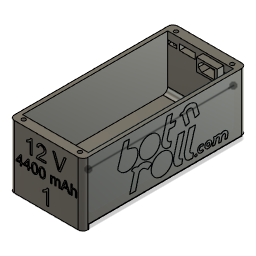
Bateria+Nova (Autodesk Fusion 360 design; units mm, degrees)
Autodesk Fusion 360 part; units mm, degrees
note: some values were not read from the file. Set by a fixed rule: which sketch regions a step uses.
sketch "Esboço1" plane through (0, 0, 0) normal (0, 1, 0) x (1, 0, 0)
  line L0 (0, 0) -> (-76, 0)
  line L1 (-76, 0) -> (-76, 169)
  line L2 (-76, 169) -> (0, 169)
  line L3 (0, 169) -> (0, 0)
  dimension "d1" = 76
  dimension "d2" = 169
  constraint horizontal L0
  constraint vertical L1
  constraint horizontal L2
  constraint vertical L3
  constraint coincident L0.start L3.end
  measures "d1" distance of L0.start L0.end
  measures "d2" distance of L0.start L2.end
extrude "Extrusão1" add sketch "Esboço1" along normal blind 65
sketch "Esboço2" plane through (0, 65, 0) normal (0, 1, 0) x (-1, 0, 0)
  line L0 (0, -169) -> (76, -169)
  line L1 (76, -169) -> (76, 0)
  line L2 (76, 0) -> (0, 0)
  line L3 (0, 0) -> (0, -169)
  line L4 (72, -159.5) -> (4, -159.5)
  line L5 (4, -159.5) -> (4, -9.5)
  line L6 (4, -9.5) -> (72, -9.5)
  line L7 (72, -9.5) -> (72, -159.5)
  dimension "d5" = 4
  dimension "d6" = 4
  dimension "d7" = 150
  dimension "d8" = 9.5
  constraint horizontal L4
  constraint vertical L5
  constraint horizontal L6
  constraint vertical L7
  measures "d5" distance of L1 L7
  measures "d6" distance of L3 L5
  measures "d7" distance of L4.start L6.end
  measures "d8" distance of L2 L6
extrude "Extrusão2" cut sketch "Esboço2" against normal blind 55 contours L4 L5 L6 L7
fillet "Arredondamento1" radius 5 2 edges at (-38, 10, -159.5) (-38, 10, -9.5)
sketch "Esboço3" plane through (-4, 0, 0) normal (-1, 0, 0) x (0, 0, 1)
  arc A0 (-14.5, 10) -> (-9.5, 15) centre (-14.5, 15) ccw
  line L0 (-9.5, 15) -> (-9.5, 65)
  line L1 (-9.5, 65) -> (-159.5, 65)
  line L2 (-159.5, 65) -> (-159.5, 15)
  arc A1 (-159.5, 15) -> (-154.5, 10) centre (-154.5, 15) ccw
  line L3 (-154.5, 10) -> (-14.5, 10)
  line L4 (-159.5, 50) -> (-155, 50)
  line L5 (-155, 50) -> (-9.5, 50)
  dimension "d13" = 40
  constraint coincident L2 L4.start
  constraint perpendicular L2 L4
  constraint coincident L0 L5.end
  constraint perpendicular L0 L5
  measures "d13" distance of L3 L5
sketch "Esboço4" plane through (0, 0, -169) normal (0, 0, -1) x (-1, 0, 0)
  line L0 (0, 0) -> (76, 0)
  line L1 (76, 0) -> (76, 65)
  line L2 (76, 65) -> (0, 65)
  line L3 (0, 65) -> (0, 0)
  line L4 (30.7398, 50) -> (35.5, 54.0801)
  line L5 (35.5, 58.9199) -> (35.5, 54.0801)
  line L6 (30.7398, 63) -> (35.5, 58.9199)
  line L7 (15, 63) -> (30.7398, 63)
  line L8 (15, 63) -> (15, 50)
  line L9 (15, 50) -> (30.7398, 50)
  line L10 (30, 52) -> (33.5, 55)
  line L11 (33.5, 58) -> (33.5, 55)
  line L12 (30, 61) -> (33.5, 58)
  line L13 (17, 61) -> (30, 61)
  line L14 (17, 52) -> (30, 52)
  line L15 (17, 61) -> (17, 52)
  line L16 (43.5, 59.5) -> (59.75, 59.5)
  line L17 (59.75, 59.5) -> (59.75, 53.5)
  line L18 (59.75, 53.5) -> (43.5, 53.5)
  line L19 (43.5, 53.5) -> (43.5, 59.5)
  dimension "d24" = 2
  dimension "d15" = 9
  dimension "d16" = 13
  dimension "d17" = 4.6098
  dimension "d18" = 3
  dimension "d19" = 4.6098
  dimension "d20" = 13
  dimension "d21" = 130.601
  dimension "d22" = 130.601
  dimension "d23" = 139.399
  dimension "d25" = 16.25
  dimension "d26" = 6
  dimension "d27" = 5.5
  dimension "d28" = 15
  dimension "d29" = 10
  dimension "d42" = 2
  constraint horizontal L16
  constraint vertical L17
  constraint horizontal L18
  constraint vertical L19
  measures "d15" distance of L14.start L13.start
  measures "d16" distance of L12.start L13.start
  measures "d17" distance of L11.start L12.start
  measures "d18" distance of L11.start L10.end
  measures "d19" distance of L10.start L10.end
  measures "d20" distance of L10.start L14.start
  measures "d21" angle of L10 L11
  measures "d22" angle of L11 L12
  measures "d23" angle of L12 L13
  measures "d25" distance of L16.start L16.end
  measures "d26" distance of L16.start L18.end
  measures "d27" distance of L2 L16
  measures "d28" distance of L3 L8
  measures "d29" distance of L11 L19
  measures "d42" distance of L2 L7
extrude "Extrusão3" cut sketch "Esboço4" against normal blind 20 contours L10 L11 L12 L13 L14 L15 | L16 L17 L18 L19
sketch "Esboço6" plane through (0, 0, -159.5) normal (0, 0, 1) x (1, 0, 0)
  line L0 (-17, 61) -> (-17, 52)
  line L1 (-17, 52) -> (-30, 52)
  line L2 (-30, 52) -> (-33.5, 55)
  line L3 (-33.5, 55) -> (-33.5, 58)
  line L4 (-33.5, 58) -> (-30, 61)
  line L5 (-30, 61) -> (-17, 61)
  line L6 (-59.75, 53.5) -> (-59.75, 59.5)
  line L7 (-59.75, 59.5) -> (-43.5, 59.5)
  line L8 (-43.5, 59.5) -> (-43.5, 53.5)
  line L9 (-43.5, 53.5) -> (-59.75, 53.5)
  line L10 (-72, 15) -> (-4, 15)
  line L11 (-4, 15) -> (-4, 65)
  line L12 (-4, 65) -> (-72, 65)
  line L13 (-72, 65) -> (-72, 15)
  line L14 (-35.5, 63) -> (-14, 63)
  line L15 (-14, 63) -> (-14, 50)
  line L16 (-14, 50) -> (-35.5, 50)
  line L17 (-35.5, 50) -> (-35.5, 63)
  dimension "d33" = 3
  dimension "d34" = 2
  dimension "d35" = 2
  dimension "d36" = 2
  constraint horizontal L14
  constraint vertical L15
  constraint horizontal L16
  constraint vertical L17
  measures "d33" distance of L0 L15
  measures "d34" distance of L5 L14
  measures "d35" distance of L3 L17
  measures "d36" distance of L1 L16
extrude "Extrusão4" add sketch "Esboço6" along normal blind 6.7 contours L14 L15 L16 L17
sketch "Esboço5" plane through (0, 0, -169) normal (0, 0, -1) x (-1, 0, 0)
  line L0 (15, 63) -> (15, 50.0001)
  line L1 (15, 50.0001) -> (30.7398, 50.0001)
  line L2 (30.7398, 50.0001) -> (35.5, 54.0802)
  line L3 (35.5, 54.0802) -> (35.5, 58.9199)
  line L4 (35.5, 58.9199) -> (30.7398, 63)
  line L5 (30.7398, 63) -> (15, 63)
  line L6 (17, 61) -> (30, 61)
  line L7 (33.5, 58) -> (33.5, 55)
extrude "Extrusão5" cut sketch "Esboço5" against normal blind 7.7
sketch "Esboço7" plane through (0, 0, -169) normal (0, 0, -1) x (-1, 0, 0)
  line L0 (15, 50.0001) -> (15, 63)
  line L1 (15, 63) -> (30.7398, 63)
  line L2 (30.7398, 63) -> (35.5, 58.9199)
  line L3 (35.5, 58.9199) -> (35.5, 54.0802)
  line L4 (35.5, 54.0802) -> (30.7398, 50.0001)
  line L5 (30.7398, 50.0001) -> (15, 50.0001)
  line L6 (59.75, 59.5) -> (59.75, 53.5)
  line L7 (59.75, 53.5) -> (43.5, 53.5)
  line L8 (43.5, 53.5) -> (43.5, 59.5)
  line L9 (43.5, 59.5) -> (59.75, 59.5)
  line L10 (0, 0) -> (76, 0)
  line L11 (76, 0) -> (76, 65)
  line L12 (76, 65) -> (0, 65)
  line L13 (0, 65) -> (0, 0)
  line L14 (0, 5) -> (76, 5)
  line L15 (4.5, 0) -> (71.5, 0)
  line L16 (4.5, 0) -> (9.5, 5)
  line L17 (71.5, 0) -> (66.5, 5)
  dimension "d43" = 5
  dimension "d45" = 57
  dimension "d46" = 45
  dimension "d47" = 45
  dimension "d48" = 4.5
  dimension "d51" = 4.5
  constraint coincident L13 L14.start
  constraint coincident L11 L14.end
  constraint perpendicular L11 L14
  constraint coincident L10 L15.start
  constraint coincident L10 L15.end
  constraint coincident L14 L16.end
  constraint coincident L14 L17.end
  measures "d43" distance of L10 L14
  measures "d45" distance of L16.end L17.end
  measures "d46" angle of L15 L16
  measures "d47" angle of L15 L17
  measures "d48" distance of L10.start L15.start
  measures "d51" distance of L10.end L15.end
extrude "Extrusão6" cut sketch "Esboço7" against normal blind 163 contours L10 L13 L14 L16 | L10 L11 L14 L17
fillet "Arredondamento2" radius 5 4 edges at (0, 35, -169) (-76, 35, -169) (0, 32.5, 0) (-76, 32.5, 0)
ref_plane "Plano de trabalho1" through (-38, 57, -84.5) normal (0, 1, 0) x (0, 0, 1)
sketch "Esboço9" plane through (-38, 57, -84.5) normal (0, 1, 0) x (1, 0, 0)
  line L0 (-26.9182, 82.6) -> (-31.3061, 82.6)
  line L1 (-33.5, 78.8) -> (-31.3061, 75)
  line L2 (-31.3061, 75) -> (-26.9182, 75)
  line L3 (-31.3061, 82.6) -> (-33.5, 78.8)
  line L4 (-24.7243, 78.8) -> (-26.9182, 82.6)
  line L5 (-26.9182, 75) -> (-24.7243, 78.8)
  line L6 (-34, 75) -> (34, 75)
  line L7 (-24.7243, 78.8) -> (-24.7243, 75)
  line L8 (-33.5, 78.8) -> (-33.5, 75)
  line L9 (-38, 79.5) -> (-38, -79.5)
  line L10 (31.3061, 75) -> (33.5, 78.8)
  line L11 (26.9182, 82.6) -> (24.7243, 78.8)
  line L12 (24.7243, 78.8) -> (26.9182, 75)
  line L13 (26.9182, 75) -> (31.3061, 75)
  line L14 (33.5, 78.8) -> (31.3061, 82.6)
  line L15 (33.5, 78.8) -> (33.5, 75)
  line L16 (24.7243, 78.8) -> (24.7243, 75)
  line L17 (31.3061, 82.6) -> (26.9182, 82.6)
  line L18 (38, -79.5) -> (38, 79.5)
  line L19 (31.3061, -75) -> (26.9182, -75)
  line L20 (24.7243, -78.8) -> (24.7243, -75)
  line L21 (26.9182, -82.6) -> (31.3061, -82.6)
  line L22 (26.9182, -75) -> (24.7243, -78.8)
  line L23 (31.3061, -82.6) -> (33.5, -78.8)
  line L24 (33.5, -78.8) -> (33.5, -75)
  line L25 (33.5, -78.8) -> (31.3061, -75)
  line L26 (24.7243, -78.8) -> (26.9182, -82.6)
  line L27 (34, -75) -> (-34, -75)
  line L28 (-31.3061, -75) -> (-33.5, -78.8)
  line L29 (-33.5, -78.8) -> (-31.3061, -82.6)
  line L30 (-24.7243, -78.8) -> (-24.7243, -75)
  line L31 (-26.9182, -82.6) -> (-24.7243, -78.8)
  line L32 (-26.9182, -75) -> (-31.3061, -75)
  line L33 (-24.7243, -78.8) -> (-26.9182, -75)
  line L34 (-31.3061, -82.6) -> (-26.9182, -82.6)
  line L35 (-33.5, -78.8) -> (-33.5, -75)
  circle A0 centre (29.1121, 78.8) radius 2
  dimension "d55" = 4.5
  dimension "d57" = 120
  dimension "d58" = 120
  dimension "d59" = 120
  dimension "d60" = 120
  dimension "d61" = 120
  dimension "d62" = 120
  dimension "d63" = 8.7757
  dimension "d64" = 4.3879
  dimension "d65" = 4.3879
  dimension "d66" = 4.3879
  dimension "d67" = 4.3879
  dimension "d68" = 4.5
  dimension "d69" = 3.8
  dimension "d70" = 3.8
  dimension "d71" = 120
  dimension "d72" = 120
  dimension "d73" = 120
  dimension "d74" = 120
  dimension "d75" = 120
  dimension "d76" = 120
  dimension "d77" = 8.7757
  dimension "d78" = 4.3879
  dimension "d79" = 4.3879
  dimension "d80" = 4.3879
  dimension "d81" = 4.3879
  dimension "d82" = 3.8
  dimension "d83" = 3.8
  dimension "d84" = 4.5
  dimension "d85" = 120
  dimension "d86" = 120
  dimension "d87" = 120
  dimension "d88" = 120
  dimension "d89" = 120
  dimension "d90" = 120
  dimension "d91" = 8.7757
  dimension "d92" = 4.3879
  dimension "d93" = 4.3879
  dimension "d94" = 4.3879
  dimension "d95" = 4.3879
  dimension "d96" = 3.8
  dimension "d97" = 3.8
  dimension "d98" = 4.5
  dimension "d101" = 4
  constraint collinear L2 L6
  constraint coincident L6 L7.end
  constraint perpendicular L6 L7
  constraint coincident L6 L8.end
  constraint perpendicular L6 L8
  constraint collinear L6 L13
  constraint collinear L19 L27
  constraint collinear L27 L32
  measures "d55" distance of L1.start L9
  measures "d57" angle of L11 L12
  measures "d58" angle of L11 L17
  measures "d59" angle of L14 L17
  measures "d60" angle of L10 L14
  measures "d61" angle of L10 L13
  measures "d62" angle of L12 L13
  measures "d63" distance of L15 L16
  measures "d64" distance of L11.end L12.end
  measures "d65" distance of L11.start L11.end
  measures "d66" distance of L11.start L14.end
  measures "d67" distance of L10.end L14.end
  measures "d68" distance of L10.end L18
  measures "d69" distance of L10.end L15.end
  measures "d70" distance of L11.end L16.end
  measures "d71" angle of L23 L25
  measures "d72" angle of L21 L23
  measures "d73" angle of L21 L26
  measures "d74" angle of L22 L26
  measures "d75" angle of L19 L22
  measures "d76" angle of L19 L25
  measures "d77" distance of L20 L24
  measures "d78" distance of L19.start L23.end
  measures "d79" distance of L21.end L23.end
  measures "d80" distance of L21.end L21.start
  measures "d81" distance of L20.start L21.start
  measures "d82" distance of L20.start L20.end
  measures "d83" distance of L23.end L24.end
  measures "d84" distance of L18 L23.end
  measures "d85" angle of L31 L33
  measures "d86" angle of L31 L34
  measures "d87" angle of L29 L34
  measures "d88" angle of L28 L29
  measures "d89" angle of L28 L32
  measures "d90" angle of L32 L33
  measures "d91" distance of L30 L35
  measures "d92" distance of L32.start L30.start
  measures "d93" distance of L31.start L30.start
  measures "d94" distance of L31.start L29.end
  measures "d95" distance of L28.end L29.end
  measures "d96" distance of L28.end L35.end
  measures "d97" distance of L30.end L30.start
  measures "d98" distance of L9 L28.end
  measures "d101" diameter of A0
extrude "Extrusão7" cut sketch "Esboço9" against normal blind 3.5 contours L0 L1 L2 L3 L4 L5 L6 | L5 L6 L7 | L1 L6 L8 | L6 L12 L16 | L6 L10 L11 L12 L13 L14 L17 | L6 L10 L15 | L19 L21 L22 L23 L25 L26 L27 | L24 L25 L27 | L20 L22 L27 | L27 L30 L33 | L27 L28 L29 L31 L32 L33 L34 | L27 L28 L35 | A0
sketch "Esboço10" plane through (0, 53.5, 0) normal (0, 1, 0) x (-1, 0, 0)
  line L0 (4.5, -163.3) -> (6.6939, -167.1)
  line L1 (6.6939, -167.1) -> (11.0818, -167.1)
  line L2 (11.0818, -167.1) -> (13.2757, -163.3)
  line L3 (13.2757, -163.3) -> (13.2757, -159.5)
  line L4 (13.2757, -159.5) -> (4.5, -159.5)
  line L5 (4.5, -159.5) -> (4.5, -163.3)
  circle A0 centre (8.8879, -163.3) radius 2
  dimension "d102" = 4
  measures "d102" diameter of A0
extrude "Extrusão8" cut sketch "Esboço10" along normal blind 15 and the other way blind 7 contours A0
sketch "Esboço11" plane through (0, 53.5, 0) normal (0, 1, 0) x (-1, 0, 0)
  line L0 (62.7243, -163.3) -> (64.9182, -167.1)
  line L1 (64.9182, -167.1) -> (69.3061, -167.1)
  line L2 (69.3061, -167.1) -> (71.5, -163.3)
  line L3 (71.5, -163.3) -> (71.5, -159.5)
  line L4 (71.5, -159.5) -> (62.7243, -159.5)
  line L5 (62.7243, -159.5) -> (62.7243, -163.3)
  circle A0 centre (67.1121, -163.3) radius 2
  dimension "d107" = 4
  measures "d107" diameter of A0
extrude "Extrusão9" cut sketch "Esboço11" along normal blind 16 and the other way blind 7 contours A0
sketch "Esboço12" plane through (0, 53.5, 0) normal (0, 1, 0) x (-1, 0, 0)
  line L0 (13.2757, -5.7) -> (11.0818, -1.9)
  line L1 (11.0818, -1.9) -> (6.6939, -1.9)
  line L2 (6.6939, -1.9) -> (4.5, -5.7)
  line L3 (4.5, -5.7) -> (4.5, -9.5)
  line L4 (4.5, -9.5) -> (13.2757, -9.5)
  line L5 (13.2757, -9.5) -> (13.2757, -5.7)
  circle A0 centre (8.8879, -5.7) radius 2
  dimension "d112" = 4
  measures "d112" diameter of A0
extrude "Extrusão10" cut sketch "Esboço12" along normal blind 14 and the other way blind 7 contours A0
sketch "Esboço13" plane through (0, 53.5, 0) normal (0, 1, 0) x (-1, 0, 0)
  line L0 (69.3061, -1.9) -> (64.9182, -1.9)
  line L1 (64.9182, -1.9) -> (62.7243, -5.7)
  line L2 (62.7243, -5.7) -> (62.7243, -9.5)
  line L3 (62.7243, -9.5) -> (71.5, -9.5)
  line L4 (71.5, -9.5) -> (71.5, -5.7)
  line L5 (71.5, -5.7) -> (69.3061, -1.9)
  circle A0 centre (67.1121, -5.7) radius 2
  dimension "d117" = 4
  measures "d117" diameter of A0
extrude "Extrusão11" cut sketch "Esboço13" along normal blind 16 and the other way blind 7 contours A0
sketch "Esboço14" plane through (0, 0, 0) normal (1, 0, 0) x (0, 0, -1)
  line L0 (5, 65) -> (5, 0)
  line L1 (5, 0) -> (6, 0)
  line L2 (6, 0) -> (6, 5)
  line L3 (6, 5) -> (164, 5)
  line L4 (164, 5) -> (164, 65)
  line L5 (164, 65) -> (5, 65)
  circle A0 centre (122.3446, 14.1582) radius 3.8205
  line L6 (48.4155, 10.0769) -> (54.4288, 10.0769)
  line L7 (87.2145, 60.5523) -> (92.5801, 60.5523)
  line L8 (93.802, 19.9229) -> (98.6495, 38.5436)
  line L9 (81.5411, 40.0726) -> (87.2145, 60.5523)
  line L10 (146.7695, 9.8868) -> (149.2547, 9.8868)
  line L11 (147.5461, 14.1582) -> (146.7695, 9.8868)
  line L12 (133.8775, 10.3139) -> (136.4404, 10.3139)
  circle A1 centre (129.6061, 14.1582) radius 3.6244
  circle A2 centre (81.6609, 20.5629) radius 11.0896
  line L13 (141.1389, 14.5854) -> (140.2847, 9.8868)
  line L14 (98.6495, 38.5436) -> (105.1538, 38.5436)
  line L15 (94.8166, 47.8472) -> (89.3362, 47.8472)
  spline S0 degree 5 poles (143.7018, 14.1582) (143.7127, 14.1735) (143.7393, 14.2074) (143.7943, 14.2681) (143.8977, 14.3689) (144.0767, 14.5273) (144.3039, 14.715) (144.5748, 14.925) (144.8809, 15.1449) (145.2085, 15.356) (145.542, 15.5369) (145.8649, 15.6666) (146.1624, 15.728) (146.4232, 15.7107) (146.6419, 15.615) (146.8205, 15.454) (146.9653, 15.248) (147.0849, 15.0207) (147.1885, 14.7951) (147.2834, 14.5881) (147.3735, 14.4091) (147.4435, 14.2919) (147.4951, 14.2192) (147.5292, 14.1774) (147.5461, 14.1582) knots 0 0 0 0 0 0 0.05 0.1 0.15 0.2 0.25 0.3 0.35 0.4 0.45 0.5 0.55 0.6 0.65 0.7 0.75 0.8 0.85 0.9 0.95 1 1 1 1 1 1
  spline S1 degree 5 poles (137.8463, 14.8833) (137.87, 14.9302) (137.9205, 15.0215) (138.0061, 15.1505) (138.1401, 15.307) (138.3407, 15.4755) (138.574, 15.6154) (138.8371, 15.7246) (139.1246, 15.8004) (139.4266, 15.8399) (139.7313, 15.84) (140.0262, 15.7978) (140.2998, 15.7107) (140.5429, 15.5774) (140.7506, 15.3982) (140.9208, 15.174) (141.0267, 14.9597) (141.0893, 14.7799) (141.1236, 14.6516) (141.1389, 14.5854) knots 0 0 0 0 0 0 0.066667 0.133333 0.2 0.266667 0.333333 0.4 0.466667 0.533333 0.6 0.666667 0.733333 0.8 0.866667 0.933333 1 1 1 1 1 1
  line L16 (142.8475, 9.8868) -> (143.7018, 14.1582)
  spline S2 degree 5 poles (87.1862, 40.0862) (87.1945, 39.9462) (87.2181, 39.6715) (87.2746, 39.2754) (87.3925, 38.7796) (87.6156, 38.2174) (87.921, 37.7174) (88.3146, 37.2844) (88.7986, 36.9199) (89.3682, 36.6204) (90.0164, 36.3805) (90.5925, 36.2322) (91.0548, 36.1438) (91.3762, 36.095) (91.5402, 36.073) knots 0 0 0 0 0 0 0.1 0.2 0.3 0.4 0.5 0.6 0.7 0.8 0.9 1 1 1 1 1 1
  line L17 (42.472, 59.8756) -> (35.8741, 38.4493)
  line L18 (53.0447, 27.2731) -> (48.4155, 10.0769)
  line L19 (114.3463, 14.3829) -> (113.4999, 9.997)
  line L20 (90.3616, 52.5439) -> (96.1177, 52.5439)
  line L21 (123.6265, 12.7419) -> (124.8156, 11.2444)
  line L22 (109.8835, 38.3897) -> (116.3878, 38.3897)
  line L23 (105.036, 19.7691) -> (109.8835, 38.3897)
  spline S3 degree 5 poles (107.0405, 54.3097) (107.0703, 54.3965) (107.1375, 54.5647) (107.2609, 54.801) (107.4713, 55.0836) (107.8114, 55.3815) (108.2274, 55.6217) (108.7141, 55.8023) (109.2596, 55.9217) (109.8439, 55.9794) (110.4429, 55.9756) (111.0311, 55.9108) (111.5846, 55.7859) (112.0839, 55.6021) (112.5177, 55.3617) (112.8808, 55.0669) (113.1138, 54.7893) (113.2566, 54.5583) (113.3376, 54.3943) (113.3746, 54.3097) knots 0 0 0 0 0 0 0.066667 0.133333 0.2 0.266667 0.333333 0.4 0.466667 0.533333 0.6 0.666667 0.733333 0.8 0.866667 0.933333 1 1 1 1 1 1
  spline S4 degree 5 poles (135.5861, 15.8668) (135.5822, 15.914) (135.5732, 16.0073) (135.5564, 16.1438) (135.5269, 16.319) (135.4778, 16.5257) (135.4152, 16.7191) (135.3378, 16.8979) (135.245, 17.0615) (135.1373, 17.2103) (135.0156, 17.3454) (134.9081, 17.4433) (134.822, 17.5114) (134.7623, 17.5544) (134.7318, 17.5754) knots 0 0 0 0 0 0 0.1 0.2 0.3 0.4 0.5 0.6 0.7 0.8 0.9 1 1 1 1 1 1
  spline S5 degree 5 poles (103.9774, 56.4454) (104.0238, 56.5789) (104.1235, 56.8411) (104.2937, 57.2208) (104.5625, 57.6994) (104.9689, 58.2505) (105.4463, 58.7516) (105.995, 59.1983) (106.6136, 59.5837) (107.299, 59.8992) (108.0463, 60.1358) (108.8479, 60.2859) (109.6934, 60.3443) (110.5688, 60.3105) (111.4574, 60.1879) (112.3416, 59.9823) (113.2044, 59.7009) (114.0306, 59.3511) (114.8091, 58.9394) (115.5334, 58.4707) (116.2001, 57.9485) (116.6866, 57.4897) (117.0252, 57.1231) (117.2394, 56.8687) (117.3435, 56.739) knots 0 0 0 0 0 0 0.05 0.1 0.15 0.2 0.25 0.3 0.35 0.4 0.45 0.5 0.55 0.6 0.65 0.7 0.75 0.8 0.85 0.9 0.95 1 1 1 1 1 1
  line L24 (105.1538, 38.5436) -> (99.5729, 18.9996)
  line L25 (100.1331, 54.3097) -> (102.696, 54.3097)
  line L26 (48.0216, 59.8756) -> (45.8859, 51.7469)
  line L27 (90.2368, 31.6712) -> (91.5402, 36.073)
  spline S6 degree 5 poles (50.1573, 30.3897) (50.2624, 30.4919) (50.4749, 30.6873) (50.8014, 30.9528) (51.252, 31.251) (51.8426, 31.5245) (52.4628, 31.6908) (53.1145, 31.7423) (53.7982, 31.6774) (54.5121, 31.5029) (55.2537, 31.2282) (55.867, 30.9353) (56.3376, 30.6772) (56.6559, 30.4883) (56.8163, 30.3897) knots 0 0 0 0 0 0 0.1 0.2 0.3 0.4 0.5 0.6 0.7 0.8 0.9 1 1 1 1 1 1
  line L28 (110.1298, 43.4973) -> (107.0405, 54.3097)
  line L29 (96.1177, 52.5439) -> (94.8166, 47.8472)
  line L30 (149.2547, 9.8868) -> (150.0313, 14.1582)
  spline S7 degree 5 poles (99.5729, 18.9996) (99.5167, 18.8712) (99.4159, 18.618) (99.2992, 18.2489) (99.2141, 17.7784) (99.2326, 17.2287) (99.3855, 16.7205) (99.6811, 16.2562) (100.1194, 15.8359) (100.6904, 15.4565) (101.3821, 15.1143) (102.0233, 14.8676) (102.5502, 14.6968) (102.9216, 14.5891) (103.1124, 14.5368) knots 0 0 0 0 0 0 0.1 0.2 0.3 0.4 0.5 0.6 0.7 0.8 0.9 1 1 1 1 1 1
  line L31 (123.6265, 15.5745) -> (125.1326, 16.7704)
  line L32 (102.266, 10.1509) -> (98.5726, 10.3048)
  spline S8 degree 5 poles (110.8069, 18.8457) (110.7507, 18.7173) (110.6498, 18.4641) (110.5332, 18.095) (110.4481, 17.6245) (110.4666, 17.0748) (110.6195, 16.5666) (110.9151, 16.1023) (111.3534, 15.682) (111.9244, 15.3026) (112.6161, 14.9604) (113.2572, 14.7137) (113.7842, 14.5429) (114.1556, 14.4352) (114.3463, 14.3829) knots 0 0 0 0 0 0 0.1 0.2 0.3 0.4 0.5 0.6 0.7 0.8 0.9 1 1 1 1 1 1
  circle A3 centre (116.7917, 10.7411) radius 1.2081
  line L33 (103.1124, 14.5368) -> (102.266, 10.1509)
  line L34 (113.4999, 9.997) -> (109.8066, 10.1509)
  line L35 (54.4288, 10.0769) -> (58.2395, 25.0247)
  line L36 (115.9375, 44.9126) -> (120.2483, 46.0882)
  line L37 (136.4404, 10.3139) -> (137.8463, 14.8833)
  spline S9 degree 5 poles (142.6176, 16.9065) (142.6864, 16.9664) (142.8269, 17.0834) (143.0457, 17.2502) (143.3537, 17.4554) (143.7658, 17.682) (144.2044, 17.8764) (144.6678, 18.0345) (145.1524, 18.1498) (145.6526, 18.2133) (146.1609, 18.2155) (146.669, 18.148) (147.168, 18.0055) (147.6487, 17.788) (148.1023, 17.5023) (148.5208, 17.1598) (148.8968, 16.7744) (149.2245, 16.3599) (149.4993, 15.9288) (149.7191, 15.4893) (149.8832, 15.0463) (149.9699, 14.6912) (150.0102, 14.4247) (150.0261, 14.247) (150.0313, 14.1582) knots 0 0 0 0 0 0 0.05 0.1 0.15 0.2 0.25 0.3 0.35 0.4 0.45 0.5 0.55 0.6 0.65 0.7 0.75 0.8 0.85 0.9 0.95 1 1 1 1 1 1
  spline S10 degree 5 poles (100.1331, 54.3097) (100.1658, 54.4044) (100.235, 54.589) (100.3505, 54.8522) (100.5285, 55.175) (100.7936, 55.5286) (101.1049, 55.828) (101.4657, 56.0693) (101.8773, 56.2509) (102.3372, 56.376) (102.8413, 56.4492) (103.2769, 56.4698) (103.6207, 56.4653) (103.8573, 56.4535) (103.9774, 56.4454) knots 0 0 0 0 0 0 0.1 0.2 0.3 0.4 0.5 0.6 0.7 0.8 0.9 1 1 1 1 1 1
  line L38 (50.1573, 30.3897) -> (53.0447, 27.2731)
  line L39 (106.1132, 42.3497) -> (110.1298, 43.4973)
  spline S11 degree 5 poles (45.8859, 51.7469) (46.0955, 51.6773) (46.5236, 51.5399) (47.1919, 51.3388) (48.1357, 51.0808) (49.398, 50.7673) (50.7261, 50.4381) (52.0863, 50.0451) (53.4198, 49.5036) (54.647, 48.709) (55.6821, 47.5773) (56.4442, 46.0778) (56.8689, 44.2705) (56.9233, 42.3439) (56.619, 40.4229) (55.9956, 38.6081) (55.1121, 36.9671) (54.0349, 35.5438) (52.8286, 34.3607) (51.5427, 33.4231) (50.211, 32.7232) (48.8561, 32.2454) (47.4932, 31.9699) (46.1337, 31.8779) (44.7893, 31.9564) (43.4731, 32.1988) (42.1977, 32.6024) (40.9745, 33.1675) (39.8125, 33.8945) (38.7175, 34.7833) (37.6925, 35.8328) (36.9295, 36.8001) (36.3893, 37.597) (36.0435, 38.1599) (35.8741, 38.4493) knots 0 0 0 0 0 0 0.033333 0.066667 0.1 0.133333 0.166667 0.2 0.233333 0.266667 0.3 0.333333 0.366667 0.4 0.433333 0.466667 0.5 0.533333 0.566667 0.6 0.633333 0.666667 0.7 0.733333 0.766667 0.8 0.833333 0.866667 0.9 0.933333 0.966667 1 1 1 1 1 1
  line L40 (56.3239, 46.2597) -> (56.8051, 44.4197)
  line L41 (66.9779, 22.9725) -> (71.5145, 26.1183)
  spline S12 degree 5 poles (105.036, 19.7691) (105.0147, 19.6377) (104.9762, 19.3713) (104.9313, 18.961) (104.897, 18.3922) (104.8982, 17.645) (104.9461, 16.8641) (105.0446, 16.0554) (105.1982, 15.2304) (105.4124, 14.4076) (105.6928, 13.609) (106.0451, 12.8577) (106.4738, 12.1747) (106.9819, 11.5765) (107.5692, 11.0713) (108.2342, 10.6618) (108.8264, 10.4106) (109.3037, 10.2645) (109.6365, 10.1857) (109.8066, 10.1509) knots 0 0 0 0 0 0 0.066667 0.133333 0.2 0.266667 0.333333 0.4 0.466667 0.533333 0.6 0.666667 0.733333 0.8 0.866667 0.933333 1 1 1 1 1 1
  line L42 (92.5801, 60.5523) -> (90.3616, 52.5439)
  spline S13 degree 5 poles (93.802, 19.9229) (93.7807, 19.7916) (93.7423, 19.5252) (93.6973, 19.1149) (93.663, 18.5461) (93.6642, 17.7989) (93.7122, 17.018) (93.8106, 16.2093) (93.9642, 15.3843) (94.1784, 14.5615) (94.4589, 13.7629) (94.8111, 13.0116) (95.2399, 12.3286) (95.7479, 11.7304) (96.3353, 11.2252) (97.0002, 10.8157) (97.5925, 10.5645) (98.0698, 10.4184) (98.4026, 10.3396) (98.5726, 10.3048) knots 0 0 0 0 0 0 0.066667 0.133333 0.2 0.266667 0.333333 0.4 0.466667 0.533333 0.6 0.666667 0.733333 0.8 0.866667 0.933333 1 1 1 1 1 1
  spline S14 degree 5 poles (137.2947, 17.5754) (137.3461, 17.5984) (137.4512, 17.6436) (137.6158, 17.7087) (137.8492, 17.7902) (138.1644, 17.8824) (138.5029, 17.9636) (138.8632, 18.0312) (139.2422, 18.081) (139.6345, 18.1075) (140.0338, 18.1045) (140.4337, 18.0657) (140.8282, 17.9859) (141.2129, 17.8617) (141.5853, 17.6921) (141.9443, 17.4775) (142.2204, 17.2706) (142.4214, 17.096) (142.5526, 16.9711) (142.6176, 16.9065) knots 0 0 0 0 0 0 0.066667 0.133333 0.2 0.266667 0.333333 0.4 0.466667 0.533333 0.6 0.666667 0.733333 0.8 0.866667 0.933333 1 1 1 1 1 1
  spline S15 degree 5 poles (134.7318, 17.5754) (134.7579, 17.6088) (134.8123, 17.6727) (134.9008, 17.7595) (135.0328, 17.8566) (135.2225, 17.9451) (135.4388, 17.9982) (135.6834, 18.0138) (135.9563, 17.9916) (136.2556, 17.9344) (136.579, 17.8453) (136.8551, 17.7508) (137.0714, 17.6677) (137.2196, 17.607) (137.2947, 17.5754) knots 0 0 0 0 0 0 0.1 0.2 0.3 0.4 0.5 0.6 0.7 0.8 0.9 1 1 1 1 1 1
  line L43 (135.5861, 15.8668) -> (133.8775, 10.3139)
  line L44 (113.3746, 54.3097) -> (115.9375, 44.9126)
  line L45 (89.3362, 47.8472) -> (87.1862, 40.0862)
  circle A4 centre (122.3446, 14.1582) radius 1.9102
  line L46 (116.3878, 38.3897) -> (110.8069, 18.8457)
  circle A5 centre (129.6061, 14.1582) radius 1.5401
  line L47 (140.2847, 9.8868) -> (142.8475, 9.8868)
  spline S16 degree 5 poles (58.2395, 25.0247) (58.3994, 25.156) (58.7204, 25.403) (59.2059, 25.7266) (59.8616, 26.0629) (60.6959, 26.3144) (61.5459, 26.384) (62.4127, 26.2599) (63.2963, 25.9415) (64.1957, 25.4418) (65.1094, 24.777) (65.8507, 24.125) (66.4122, 23.5729) (66.7889, 23.1772) (66.9779, 22.9725) knots 0 0 0 0 0 0 0.1 0.2 0.3 0.4 0.5 0.6 0.7 0.8 0.9 1 1 1 1 1 1
  spline S17 degree 5 poles (87.1862, 40.0862) (87.1945, 39.9462) (87.2181, 39.6715) (87.2746, 39.2754) (87.3925, 38.7796) (87.6156, 38.2174) (87.921, 37.7174) (88.3146, 37.2844) (88.7986, 36.9199) (89.3682, 36.6204) (90.0164, 36.3805) (90.5925, 36.2322) (91.0548, 36.1438) (91.3762, 36.095) (91.5402, 36.073) knots 0 0 0 0 0 0 0.1 0.2 0.3 0.4 0.5 0.6 0.7 0.8 0.9 1 1 1 1 1 1
  line L48 (42.472, 59.8756) -> (48.0216, 59.8756)
  circle A6 centre (69.0872, 42.5633) radius 10.8261
  line L49 (120.2483, 46.0882) -> (117.3435, 56.739)
  line L50 (102.696, 54.3097) -> (106.1132, 42.3497)
  spline S18 degree 5 poles (81.5411, 40.0726) (81.5269, 39.9099) (81.5078, 39.584) (81.5073, 39.0931) (81.5633, 38.4346) (81.7299, 37.6059) (81.9954, 36.7753) (82.361, 35.9499) (82.8248, 35.1428) (83.3809, 34.3729) (84.0215, 33.6621) (84.7379, 33.0326) (85.5212, 32.5042) (86.3639, 32.0908) (87.2596, 31.7981) (88.2037, 31.6271) (88.9952, 31.5861) (89.6084, 31.6083) (90.0259, 31.6464) (90.2368, 31.6712) knots 0 0 0 0 0 0 0.066667 0.133333 0.2 0.266667 0.333333 0.4 0.466667 0.533333 0.6 0.666667 0.733333 0.8 0.866667 0.933333 1 1 1 1 1 1
  spline S19 degree 5 poles (56.8163, 30.3897) (56.9499, 30.5004) (57.2258, 30.7107) (57.6653, 30.9925) (58.3029, 31.3002) (59.1868, 31.569) (60.1555, 31.7186) (61.2021, 31.7466) (62.3107, 31.6535) (63.4584, 31.4425) (64.6191, 31.118) (65.7665, 30.6854) (66.8775, 30.1503) (67.9356, 29.5189) (68.9324, 28.7972) (69.864, 27.9906) (70.5566, 27.2807) (71.0469, 26.7131) (71.3608, 26.3191) (71.5145, 26.1183) knots 0 0 0 0 0 0 0.066667 0.133333 0.2 0.266667 0.333333 0.4 0.466667 0.533333 0.6 0.666667 0.733333 0.8 0.866667 0.933333 1 1 1 1 1 1
  point P0 (93.802, 16.3555)
  point P1 (110.8069, 16.3065)
  point P2 (106.4979, 12.19)
  point P3 (95.264, 12.3439)
  point P4 (105.036, 16.2017)
  point P5 (135.3241, 16.9137)
  point P6 (140.7118, 18.0028)
  point P7 (41.0119, 33.196)
  point P8 (149.2547, 16.2939)
  point P9 (56.5645, 45.3397)
  point P10 (147.119, 18.0028)
  point P11 (60.5102, 31.7109)
  point P12 (135.5861, 18.0025)
  point P13 (99.5729, 16.4604)
  point P14 (90.8885, 41.3514)
  point P15 (51.294, 50.2622)
  point P16 (138.8033, 15.7024)
  point P17 (62.0791, 26.2825)
  point P18 (146.3545, 15.7024)
  point P19 (46.9537, 31.9567)
  point P20 (144.602, 18.0028)
  point P21 (88.2612, 37.3728)
  point P22 (140.2847, 15.7024)
  point P23 (66.349, 30.3897)
  point P24 (144.5247, 14.8833)
  point P25 (105.7134, 58.9547)
  point P26 (53.5484, 35.1128)
  point P27 (52.9436, 31.7109)
  point P28 (88.2612, 37.3728)
  point P29 (138.726, 18.0028)
  point P30 (101.4146, 56.0183)
  point P31 (111.666, 55.7421)
  point P32 (85.3803, 32.6258)
  point P33 (147.1474, 14.8833)
  point P34 (109.1032, 60.2897)
  point P35 (113.8017, 59.4354)
  point P36 (82.2721, 36.1861)
  point P37 (108.5852, 55.7421)
  constraint horizontal L7
  constraint parallel L9 L42
  constraint parallel L7 L20
  constraint parallel L9 L29
  constraint parallel L15 L20
  constraint parallel L29 L45
  constraint horizontal L25
  constraint perpendicular L39 L50
  constraint perpendicular L28 L39
  constraint perpendicular L36 L44
  constraint perpendicular L36 L49
  constraint horizontal L6
  constraint horizontal L14
  constraint horizontal L22
  constraint concentric A0 A4
  constraint coincident L21.start A4
  constraint coincident L21.end A0
  constraint coincident L31.start A4
  constraint coincident L31.end A0
  constraint perpendicular L21 L31
  constraint concentric A1 A5
  constraint horizontal L12
  constraint parallel L37 L43
  constraint horizontal L47
  constraint parallel L11 L13
  constraint parallel L10 L47
  constraint parallel L11 L30
  constraint horizontal L48
  constraint midpoint P9 L40
extrude "Extrusão12" cut sketch "Esboço14" against normal blind 0.2 contours A0 L21 L31 A4 | A0 A1 | L6 L18 S6 L35 L38 L41 S16 S19 | L7 L9 L15 S2 L20 L27 L29 L42 L45 S17 S18 | L8 L14 L24 S7 L32 L33 S13 | L10 L11 L12 L13 S0 S1 L16 S4 L30 L37 S9 S14 S15 L43 L47 | A2 | L17 L26 S11 L48 | L19 L22 L23 S8 L34 S12 L46 | S3 S5 L25 L28 L36 S10 L39 L44 L49 L50 | A3 | A6 picked at (126.8307, 14.9343)
sketch "Esboço15" plane through (-76, 0, 0) normal (-1, 0, 0) x (0, 0, 1)
  line L0 (-5, 0) -> (-5, 65)
  line L1 (-5, 65) -> (-164, 65)
  line L2 (-164, 65) -> (-164, 5)
  line L3 (-164, 5) -> (-6, 5)
  line L4 (-6, 5) -> (-6, 0)
  line L5 (-6, 0) -> (-5, 0)
  arc A0 (-86.8867, 11.9907) -> (-83.4362, 10.8714) centre (-85.1614, 11.431) ccw
  line L6 (-110.1523, 44.4106) -> (-128.871, 44.4106)
  line L7 (-91.886, 12.5263) -> (-107.0162, 12.5263)
  line L8 (-110.1523, 42.7671) -> (-128.871, 42.7671) construction
  line L9 (-107.0162, 60.184) -> (-107.0162, 53.4594) construction
  arc A1 (-62.9503, 10.554) -> (-59.2688, 10.554) centre (-61.1095, 10.554) ccw
  line L10 (-54.9009, 38.2079) -> (-61.1095, 38.2079)
  arc A2 (-110.1523, 41.1236) -> (-110.1523, 44.4106) centre (-110.1523, 42.7671) ccw
  line L11 (-116.1476, 36.3187) -> (-126.7215, 30.6419)
  line L12 (-99.1506, 34.491) -> (-89.8244, 29.0114) construction
  line L13 (-100.2335, 32.6479) -> (-90.9073, 27.1684)
  arc A3 (-109.0674, 53.4594) -> (-104.9651, 53.4594) centre (-107.0162, 53.4594) ccw
  line L14 (-108.6135, 36.6481) -> (-108.6135, 17.0624)
  arc A4 (-126.7215, 30.6419) -> (-125.2701, 27.9385) centre (-125.9958, 29.2902) ccw
  arc A5 (-105.4189, 36.6481) -> (-108.6135, 36.6481) centre (-107.0162, 36.6481) ccw
  line L15 (-105.4189, 17.0624) -> (-105.4189, 36.6481)
  arc A6 (-98.0678, 36.334) -> (-100.2335, 32.6479) centre (-99.1506, 34.491) ccw
  arc A7 (-107.0162, 12.5263) -> (-107.0162, 9.3707) centre (-107.0162, 10.9485) ccw
  arc A8 (-128.871, 44.4106) -> (-128.871, 41.1236) centre (-128.871, 42.7671) ccw
  line L16 (-103.2495, 42.7013) -> (-84.5133, 42.7013) construction
  arc A9 (-103.2495, 44.4763) -> (-103.2495, 40.9263) centre (-103.2495, 42.7013) ccw
  arc A10 (-114.6962, 33.6152) -> (-116.1476, 36.3187) centre (-115.4219, 34.9669) ccw
  line L17 (-107.0162, 36.6481) -> (-107.0162, 17.0624) construction
  arc A11 (-108.6135, 17.0624) -> (-105.4189, 17.0624) centre (-107.0162, 17.0624) ccw
  arc A12 (-75.0746, 13.1122) -> (-75.0746, 17.3307) centre (-75.0746, 15.2214) ccw
  arc A13 (-91.886, 9.3707) -> (-91.886, 12.5263) centre (-91.886, 10.9485) ccw
  line L18 (-103.2495, 40.9263) -> (-84.5133, 40.9263)
  line L19 (-107.0162, 9.3707) -> (-91.886, 9.3707)
  line L20 (-104.9651, 53.4594) -> (-104.9651, 60.184)
  line L21 (-125.9958, 29.2902) -> (-115.4219, 34.9669) construction
  line L22 (-125.2701, 27.9385) -> (-114.6962, 33.6152)
  line L23 (-109.0674, 60.184) -> (-109.0674, 53.4594)
  line L24 (-107.0162, 10.9485) -> (-91.886, 10.9485) construction
  line L25 (-128.871, 41.1236) -> (-110.1523, 41.1236)
  line L26 (-84.5133, 44.4763) -> (-103.2495, 44.4763)
  arc A14 (-104.9651, 60.184) -> (-109.0674, 60.184) centre (-107.0162, 60.184) ccw
  line L27 (-88.7415, 30.8545) -> (-98.0678, 36.334)
  line L28 (-83.9319, 13.1122) -> (-75.0746, 13.1122)
  line L29 (-48.168, 11.5257) -> (-53.3151, 20.783)
  arc A15 (-69.0853, 9.9398) -> (-66.1505, 10.9053) centre (-67.6179, 10.4225) ccw
  arc A16 (-75.4251, 35.5676) -> (-78.8756, 36.6869) centre (-77.1503, 36.1272) ccw
  line L30 (-62.9503, 30.2763) -> (-62.9503, 10.554)
  arc A17 (-84.5133, 40.9263) -> (-84.5133, 44.4763) centre (-84.5133, 42.7013) ccw
  line L31 (-75.0746, 17.3307) -> (-83.9319, 17.3307)
  line L32 (-66.1505, 10.9053) -> (-72.7904, 31.0878)
  line L33 (-59.2688, 10.554) -> (-59.2688, 30.2763)
  arc A18 (-83.9319, 17.3307) -> (-83.9319, 13.1122) centre (-83.9319, 15.2214) ccw
  line L34 (-74.2577, 30.605) -> (-67.6179, 10.4225) construction
  line L35 (-55.0631, 19.8111) -> (-49.916, 10.5538) construction
  arc A19 (-54.9009, 34.9669) -> (-54.9009, 38.2079) centre (-54.9009, 36.5874) ccw
  line L36 (-78.8756, 36.6869) -> (-86.8867, 11.9907)
  line L37 (-61.1095, 34.9669) -> (-54.9009, 34.9669)
  arc A20 (-53.3151, 20.783) -> (-56.8111, 18.8392) centre (-55.0631, 19.8111) ccw
  arc A21 (-72.7904, 31.0878) -> (-75.7251, 30.1223) centre (-74.2577, 30.605) ccw
  line L38 (-75.7251, 30.1223) -> (-69.0853, 9.9398)
  line L39 (-61.1095, 30.2763) -> (-61.1095, 10.554) construction
  arc A22 (-61.1095, 38.2079) -> (-61.1095, 34.9669) centre (-61.1095, 36.5874) ccw
  line L40 (-85.1614, 11.431) -> (-77.1503, 36.1272) construction
  arc A23 (-54.8872, 21.8009) -> (-54.9377, 17.8146) centre (-54.9124, 19.8077) ccw
  arc A24 (-90.9073, 27.1684) -> (-88.7415, 30.8545) centre (-89.8244, 29.0114) ccw
  line L41 (-83.4362, 10.8714) -> (-75.4251, 35.5676)
  line L42 (-83.9319, 15.2214) -> (-75.0746, 15.2214) construction
  arc A25 (-54.8872, 21.8009) -> (-51.1291, 31.8208) centre (-54.8151, 27.4886) ccw
  arc A26 (-48.5457, 34.8571) -> (-51.1291, 31.8208) centre (-49.8374, 33.3389) ccw
  arc A27 (-51.664, 9.582) -> (-48.168, 11.5257) centre (-49.916, 10.5538) ccw
  line L43 (-56.8111, 18.8392) -> (-51.664, 9.582)
  line L44 (-61.1095, 36.5874) -> (-54.9009, 36.5874) construction
  arc A28 (-54.9377, 17.8146) -> (-48.5457, 34.8571) centre (-54.8151, 27.4886) ccw
  arc A29 (-54.9124, 19.8077) -> (-49.8374, 33.3389) centre (-54.8151, 27.4886) ccw construction
  arc A30 (-59.2688, 30.2763) -> (-62.9503, 30.2763) centre (-61.1095, 30.2763) ccw
  point P0 (-114.8899, 13.1238)
  dimension "d124" = 2
  constraint tangent A3 L23
  constraint tangent A3 L20
  constraint parallel L20 L23
  constraint tangent L20 A14
  constraint tangent L23 A14
  constraint tangent L18 A17
  constraint tangent L26 A17
  constraint parallel L18 L26
  constraint tangent A9 L26
  constraint tangent A9 L18
  constraint tangent L13 A24
  constraint tangent L27 A24
  constraint parallel L13 L27
  constraint tangent A6 L27
  constraint tangent L13 A6
  constraint tangent L14 A11
  constraint tangent L15 A11
  constraint parallel L14 L15
  constraint tangent A5 L15
  constraint tangent L14 A5
  constraint tangent A10 L22
  constraint tangent L11 A10
  constraint parallel L11 L22
  constraint tangent L11 A4
  constraint tangent A4 L22
  constraint tangent L6 A8
  constraint tangent A8 L25
  constraint parallel L6 L25
  constraint tangent A2 L25
  constraint tangent L6 A2
  constraint perpendicular L8 L14
  constraint tangent A13 L19
  constraint tangent L7 A13
  constraint parallel L7 L19
  constraint tangent L7 A7
  constraint tangent A7 L19
  constraint perpendicular L14 L24
  constraint tangent A16 L41
  constraint tangent A16 L36
  constraint parallel L36 L41
  constraint tangent A0 L36
  constraint tangent A0 L41
  constraint tangent A12 L28
  constraint tangent A12 L31
  constraint parallel L28 L31
  constraint tangent L31 A18
  constraint tangent L28 A18
  constraint coincident A18.centre L40
  constraint tangent A15 L38
  constraint tangent A15 L32
  constraint parallel L32 L38
  constraint tangent L32 A21
  constraint tangent A21 L38
  constraint tangent A1 L30
  constraint tangent A1 L33
  constraint parallel L30 L33
  constraint tangent L33 A30
  constraint tangent L30 A30
  constraint tangent A19 L37
  constraint tangent L10 A19
  constraint parallel L10 L37
  constraint tangent L10 A22
  constraint tangent L37 A22
  constraint tangent A23 A28
  constraint tangent A23 A25
  constraint tangent A25 A26
  constraint tangent A26 A28
  constraint tangent A27 L43
  constraint tangent L29 A27
  constraint parallel L29 L43
  constraint tangent L29 A20
  constraint tangent A20 L43
  constraint coincident L35.start A29
  measures "d124" radius of A27
extrude "Extrusão13" cut sketch "Esboço15" against normal blind 0.2 contours A0 L28 A18 L36 L41 | L28 L31 A18 L36 L41 | A18 L36 | A12 L28 L31 L41 | A16 L31 A18 L36 L41 | L6 A2 A8 L25 | L7 A7 A13 L19 | A1 L30 L33 A30 | L10 A19 L37 A22 | L11 A4 A10 L22 | L13 A6 L27 A24 | A3 L20 L23 A14 | L14 A5 L15 A11 | A9 L18 L26 A17 | L29 A20 A23 A25 A27 L43 A28 | L29 A20 A23 A25 A28 | L29 A20 A25 A26 A28 | A15 L32 A21 L38
sketch "Esboço16" plane through (0, 0, 0) normal (0, 0, 1) x (1, 0, 0)
  line L0 (-71, 65) -> (-71, 0)
  line L1 (-71, 0) -> (-5, 0)
  line L2 (-5, 0) -> (-5, 65)
  line L3 (-5, 65) -> (-71, 65)
  line L4 (-71, 32.5) -> (-5, 32.5) construction
  line L5 (-5, 32.5) -> (-5, 67.5) construction
  line L6 (-5, 67.5) -> (-71, 67.5) construction
  line L7 (-71, 67.5) -> (-71, 32.5) construction
  line L8 (-71, -1804.8404) -> (-5, -1804.8404) construction
  line L9 (-5, -1804.8404) -> (-5, 1869.8404) construction
  line L10 (-5, 1869.8404) -> (-71, 1869.8404) construction
  line L11 (-71, 1869.8404) -> (-71, -1804.8404) construction
  line L12 (-59.7382, 6.7597) -> (-17.7382, 6.7597) construction
  line L13 (-17.7382, 6.7597) -> (-17.7382, 19.9839) construction
  line L14 (-17.7382, 19.9839) -> (-59.7382, 19.9839) construction
  line L15 (-59.7382, 19.9839) -> (-59.7382, 6.7597) construction
  dimension "d313" = 15
  dimension "d314" = 10
  dimension "d317" = 16
  text T0 "12 V" font "Arial" height 15 align centre middle in box 66 x 35 at (-71, 32.5) x (1, 0) y (0, 1) spacing 1
  text T1 "4400 mAh" font "Arial" height 10 align centre middle in box 66 x 3674.6808 at (-71, -1804.8404) x (1, 0) y (0, 1) spacing 1
  text T2 "1" font "Arial" height 16 align centre middle in box 42 x 13.2243 at (-59.7382, 6.7597) x (1, 0) y (0, 1) spacing 1
  constraint coincident L7
  constraint midpoint L2
  constraint coincident L2
  constraint coincident L9
extrude "Extrusão14" cut sketch "Esboço16" against normal blind 0.3 text T2 T1 T0
